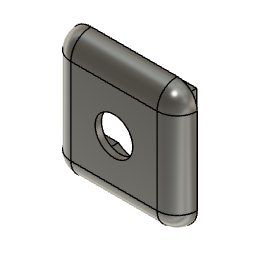
Back Plate (Autodesk Fusion 360 design; units mm, degrees)
Autodesk Fusion 360 part; units mm, degrees
note: some values were not read from the file. Set by a fixed rule: which sketch regions a step uses.
sketch "Sketch1" plane through (0, 0, 0) normal (0, 1, 0) x (1, 0, 0)
  line L0 (0, 0) -> (69.24, 0)
  line L1 (69.24, 0) -> (69.24, -69.24)
  line L2 (69.24, -69.24) -> (0, -69.24)
  line L3 (0, -69.24) -> (0, 0)
  dimension "d1" = 69.24
  dimension "d2" = 69.24
  constraint horizontal L0
  constraint vertical L1
  constraint horizontal L2
  constraint vertical L3
  constraint coincident L0.start L3.end
  measures "d1" distance of L0.start L0.end
  measures "d2" distance of L0.start L2.end
extrude "Extrude1" add sketch "Sketch1" along normal blind 5.08
sketch "Sketch2" plane through (0, 0, 0) normal (0, -1, 0) x (1, 0, 0)
  line L0 (69.24, 69.24) -> (0, 69.24)
  line L1 (0, 69.24) -> (0, 0)
  line L2 (0, 0) -> (69.24, 0)
  line L3 (69.24, 0) -> (69.24, 69.24)
  line L4 (-5.38, 74.62) -> (74.62, 74.62)
  line L5 (74.62, 74.62) -> (74.62, -5.38)
  line L6 (74.62, -5.38) -> (-5.38, -5.38)
  line L7 (-5.38, -5.38) -> (-5.38, 74.62)
  point P0 (34.62, 69.24)
  point P1 (34.62, 74.62)
  point P2 (0, 34.62)
  point P3 (-5.38, 34.62)
  dimension "d5" = 80
  dimension "d6" = 80
  constraint horizontal L4
  constraint vertical L5
  constraint horizontal L6
  constraint vertical L7
  constraint midpoint L0 P0
  constraint midpoint L4 P1
  constraint vertical P0 P1
  constraint midpoint L1 P2
  constraint midpoint L7 P3
  constraint horizontal P2 P3
  measures "d5" distance of L4.start L4.end
  measures "d6" distance of L4.start L6.end
extrude "Extrude2" add sketch "Sketch2" along normal blind 12.7 contours L0 L1 L2 L3 | L4 L5 L6 L7
fillet "Fillet1" radius 12.7 8 edges at (-5.38, -6.35, 74.62) (74.62, -6.35, 74.62) (74.62, -6.35, -5.38) (-5.38, -6.35, -5.38) (34.62, -12.7, 74.62) (-5.38, -12.7, 34.62) (74.62, -12.7, 34.62) (34.62, -12.7, -5.38)
sketch "Sketch4" plane through (0, -12.7, 0) normal (0, -1, 0) x (1, 0, 0)
  line L0 (7.32, 7.32) -> (61.92, 7.32)
  line L1 (61.92, 7.32) -> (61.92, 61.92)
  line L2 (61.92, 61.92) -> (7.32, 61.92)
  line L3 (7.32, 61.92) -> (7.32, 7.32)
  circle A0 centre (34.62, 34.62) radius 11.938
  dimension "d18" = 23.876
  measures "d18" diameter of A0
extrude "Extrude4" cut sketch "Sketch4" against normal up to surface (17.78 mm away) contours A0
sketch "Sketch5" plane through (0, 5.08, 0) normal (0, 1, 0) x (-1, 0, 0)
  circle A0 centre (-34.62, 34.62) radius 11.938
  line L0 (0, 69.24) -> (-69.24, 69.24)
  line L1 (-69.24, 69.24) -> (-69.24, 0)
  line L2 (-69.24, 0) -> (0, 0)
  line L3 (0, 0) -> (0, 69.24)
  circle A1 centre (-34.62, 34.62) radius 25
  line L4 (-69.24, 54.62) -> (0, 54.62)
  line L5 (0, 54.62) -> (0, 14.62)
  line L6 (0, 14.62) -> (-69.24, 14.62)
  line L7 (-69.24, 14.62) -> (-69.24, 54.62)
  line L8 (-69.24, 54.62) -> (0, 14.62) construction
  line L9 (0, 54.62) -> (-69.24, 14.62) construction
  point P0 (-34.62, 34.62)
  dimension "d21" = 50
  dimension "d24" = 40
  constraint concentric A0 A1
  constraint horizontal L4
  constraint perpendicular L4 L5
  constraint parallel L4 L6
  constraint parallel L5 L7
  constraint coincident L8 P0
  constraint coincident L9 P0
  constraint coincident P0 A0.centre
  measures "d21" diameter of A1
  measures "d24" distance of L4.end L5.end
extrude "Extrude5" cut sketch "Sketch5" against normal blind 13.78 contours L3 A1 L4 L5 L6 | L1 A1 L4 L6 L7 | A1 L4 | A1 L4 L6 | A1 L6
ref_plane "WorkPlane2" through (34.62, 2.54, -7.62) normal (0, 0, -1) x (-1, 0, 0)
sketch "Sketch7" plane through (0, 0, -7.62) normal (0, 0, -1) x (-1, 0, 0)
  line L0 (-61.92, 0) -> (-7.32, 0)
  circle A0 centre (-34.62, 0) radius 5.08
  dimension "d28" = 10.16
  constraint midpoint L0 A0.centre
  measures "d28" diameter of A0
extrude "Extrude6" cut sketch "Sketch7" against normal blind 5.08 contours L0 A0 picked at (-34.2432, -1.6509)
equation "d1 = 8 cm - 0.4 in - 0.6 mm"
equation "d2 = 8 cm - 0.4 in - 0.6 mm"
equation "d22 = -( 0.7 in - 0.4 cm )"
